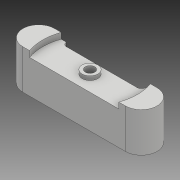
# Autodesk Inventor part: phalanx_1_gearbox_support
Saved by Autodesk Inventor 2017 SP1 (Build 210196100, 196)
## iProperties
Created: 2018-01-05
Part Number: phalanx_1_gearbox_support
Material: Generic
Document SubType Name: Modeling
Designer: JT
Density: 1 g/cm^3
Appearance: Default
Author: JT
Autodesk Inventor part; units mm, degrees
ref_plane "YZ Plane" through (0, 0, 0) normal (1, 0, 0) x (0, 1, 0)
ref_plane "XZ Plane" through (0, 0, 0) normal (0, 1, 0) x (-1, 0, 0)
ref_plane "XY Plane" through (0, 0, 0) normal (0, 0, 1) x (1, 0, 0)
sketch "Sketch1" plane through (0, 0, 0) normal (0, 0, 1) x (1, 0, 0)
  line L0 (-6.5, 0) -> (6.5, 0) construction
  line L1 (-6.5, -2) -> (6.5, -2)
  line L2 (6.5, 2) -> (-6.5, 2)
  arc A0 (-6.5, 2) -> (-6.5, -2) centre (-6.5, 0) ccw
  arc A1 (6.5, -2) -> (6.5, 2) centre (6.5, 0) ccw
  point P0 (0, 0)
  dimension "d0" = 17
  dimension "d1" = 4
  constraints: 8 end point, 4 point on circle, 4 tangent, 2 centre point, 1 horizontal, 1 midpoint, 1 parallel
  measures "d1" distance between parallel lines of L1 L2
extrude "Extrusion1" add sketch "Sketch1" along normal blind 5
sketch "Sketch2" plane through (0, 0, 5) normal (0, 0, 1) x (1, 0, 0)
  circle A0 centre (0, 0) radius 6
  dimension "d4" = 12
  constraints: 1 centre point, 1 coincident
  measures "d4" diameter of A0
extrude "Extrusion2" cut sketch "Sketch2" against normal blind 0.75
sketch "Sketch3" plane through (0, 0, 4.25) normal (0, 0, 1) x (1, 0, 0)
  circle A0 centre (0, 0) radius 1
  dimension "d7" = 2
  constraints: 1 centre point, 1 coincident
  measures "d7" diameter of A0
extrude "Extrusion3" add sketch "Sketch3" along normal blind 0.5
hole "Hole1" at (0, 0, 4.75) direction (0, 0, -1) diameter 1.2 depth 3.3 tip angle 118
sketch "Sketch4" plane through (0, 0, 0) normal (0, 0, -1) x (-1, 0, 0)
  line L0 (6.5, -2) -> (-6.5, -2) projected
  arc A0 (6.5, -2) -> (6.5, 2) centre (6.5, 0) ccw projected
  line L1 (-6.5, 2) -> (6.5, 2) projected
  arc A1 (-6.5, 2) -> (-6.5, -2) centre (-6.5, 0) ccw projected
  line L2 (-4.5, 2) -> (4.5, 2) construction
  line L3 (-6.5, 2) -> (6.5, 2) projected
  line L4 (-4.5, 1.5) -> (4.5, 1.5)
  line L5 (4.5, 2.5) -> (-4.5, 2.5)
  arc A2 (-4.5, 2.5) -> (-4.5, 1.5) centre (-4.5, 2) ccw
  arc A3 (4.5, 1.5) -> (4.5, 2.5) centre (4.5, 2) ccw
  point P0 (0, 0)
  point P1 (0, 2)
  point P2 (0, 2)
  dimension "d19" = 0.5
  dimension "d20" = 10
  constraints: 8 end point, 4 point on circle, 4 tangent, 2 centre point, 2 midpoint, 2 point on line, 1 coincident, 1 parallel
  measures "d19" distance between parallel lines of L4 L1
extrude "Extrusion4" cut sketch "Sketch4" against normal through all contours A3 L4 A2 L1 | L1 A2 L5 A3
body "Solid1"
